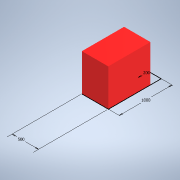
# Autodesk Inventor part: 桌1
Saved by Autodesk Inventor 2020 (Build 240168000, 168)
## iProperties
Created: 2023-03-07
Part Number: 桌1
Material: 一般
Document SubType Name: Modeling
Designer: robot
Density: 1 g/cm^3
Appearance: 銅 - 緞
Mass: 280000 g
Surface Area: 26200 cm^2
Volume: 280000 cm^3
Author: robot
Autodesk Inventor part; units mm, degrees
ref_plane "YZ Plane" through (0, 0, 0) normal (1, 0, 0) x (0, 1, 0)
ref_plane "XZ Plane" through (0, 0, 0) normal (0, 1, 0) x (-1, 0, 0)
ref_plane "XY Plane" through (0, 0, 0) normal (0, 0, 1) x (1, 0, 0)
sketch "草圖1" plane through (0, 0, 0) normal (0, 1, 0) x (-1, 0, 0)
  line L0 (0, 0) -> (500, 0)
  line L1 (500, -800) -> (0, -800)
  line L2 (500, -800) -> (500, 0)
  line L3 (0, -800) -> (0, 0)
  line L4 (500, 0) -> (0, 0)
  constraints: 10 end point, 1 collinear, 1 horizontal, 1 perpendicular, 1 vertical
extrude "擠出1" add sketch "草圖1" along normal blind 700
